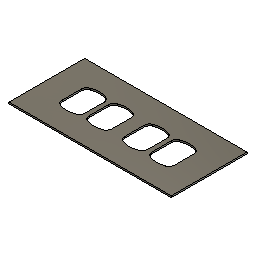
NixieClockFront (Autodesk Fusion 360 design; units mm, degrees)
Autodesk Fusion 360 part; units mm, degrees
sketch "Skizze1" plane through (0, 0, 0) normal (0, 1, 0) x (1, 0, 0)
  line L0 (-60, 12.25) -> (-60, -12.25)
  line L1 (-60, -12.25) -> (-81, -12.25) construction
  line L2 (-81, -12.25) -> (-81, 12.25)
  line L3 (-35, 12.25) -> (-35, -12.25)
  line L4 (-35, -12.25) -> (-56, -12.25) construction
  line L5 (-56, -12.25) -> (-56, 12.25)
  line L6 (-2, 12.25) -> (-2, -12.25)
  line L7 (-2, -12.25) -> (-23, -12.25) construction
  line L8 (-23, -12.25) -> (-23, 12.25)
  line L9 (23, 12.25) -> (23, -12.25)
  line L10 (23, -12.25) -> (2, -12.25) construction
  line L11 (2, -12.25) -> (2, 12.25)
  spline S0 degree 5 poles (-81, 12.25) (-80.58, 12.4586) (-79.74, 12.8575) (-78.48, 13.4013) (-76.8, 14.0152) (-74.7, 14.5849) (-72.6, 14.9392) (-70.5, 15.0605) (-68.4, 14.9392) (-66.3, 14.5849) (-64.2, 14.0152) (-62.52, 13.4013) (-61.26, 12.8575) (-60.42, 12.4586) (-60, 12.25) knots 0 0 0 0 0 0 0.1 0.2 0.3 0.4 0.5 0.6 0.7 0.8 0.9 1 1 1 1 1 1
  spline S1 degree 5 poles (-56, 12.25) (-55.58, 12.4586) (-54.74, 12.8575) (-53.48, 13.4013) (-51.8, 14.0152) (-49.7, 14.5849) (-47.6, 14.9392) (-45.5, 15.0605) (-43.4, 14.9392) (-41.3, 14.5849) (-39.2, 14.0152) (-37.52, 13.4013) (-36.26, 12.8575) (-35.42, 12.4586) (-35, 12.25) knots 0 0 0 0 0 0 0.1 0.2 0.3 0.4 0.5 0.6 0.7 0.8 0.9 1 1 1 1 1 1
  spline S2 degree 5 poles (-23, 12.25) (-22.58, 12.4586) (-21.74, 12.8575) (-20.48, 13.4013) (-18.8, 14.0152) (-16.7, 14.5849) (-14.6, 14.9392) (-12.5, 15.0605) (-10.4, 14.9392) (-8.3, 14.5849) (-6.2, 14.0152) (-4.52, 13.4013) (-3.26, 12.8575) (-2.42, 12.4586) (-2, 12.25) knots 0 0 0 0 0 0 0.1 0.2 0.3 0.4 0.5 0.6 0.7 0.8 0.9 1 1 1 1 1 1
  spline S3 degree 5 poles (2, 12.25) (2.42, 12.4586) (3.26, 12.8575) (4.52, 13.4013) (6.2, 14.0152) (8.3, 14.5849) (10.4, 14.9392) (12.5, 15.0605) (14.6, 14.9392) (16.7, 14.5849) (18.8, 14.0152) (20.48, 13.4013) (21.74, 12.8575) (22.58, 12.4586) (23, 12.25) knots 0 0 0 0 0 0 0.1 0.2 0.3 0.4 0.5 0.6 0.7 0.8 0.9 1 1 1 1 1 1
  spline S4 degree 5 poles (-81, -12.25) (-80.58, -12.4586) (-79.74, -12.8575) (-78.48, -13.4013) (-76.8, -14.0152) (-74.7, -14.5849) (-72.6, -14.9392) (-70.5, -15.0605) (-68.4, -14.9392) (-66.3, -14.5849) (-64.2, -14.0152) (-62.52, -13.4013) (-61.26, -12.8575) (-60.42, -12.4586) (-60, -12.25) knots 0 0 0 0 0 0 0.1 0.2 0.3 0.4 0.5 0.6 0.7 0.8 0.9 1 1 1 1 1 1
  spline S5 degree 5 poles (-56, -12.25) (-55.58, -12.4586) (-54.74, -12.8575) (-53.48, -13.4013) (-51.8, -14.0152) (-49.7, -14.5849) (-47.6, -14.9392) (-45.5, -15.0605) (-43.4, -14.9392) (-41.3, -14.5849) (-39.2, -14.0152) (-37.52, -13.4013) (-36.26, -12.8575) (-35.42, -12.4586) (-35, -12.25) knots 0 0 0 0 0 0 0.1 0.2 0.3 0.4 0.5 0.6 0.7 0.8 0.9 1 1 1 1 1 1
  spline S6 degree 5 poles (-23, -12.25) (-22.58, -12.4586) (-21.74, -12.8575) (-20.48, -13.4013) (-18.8, -14.0152) (-16.7, -14.5849) (-14.6, -14.9392) (-12.5, -15.0605) (-10.4, -14.9392) (-8.3, -14.5849) (-6.2, -14.0152) (-4.52, -13.4013) (-3.26, -12.8575) (-2.42, -12.4586) (-2, -12.25) knots 0 0 0 0 0 0 0.1 0.2 0.3 0.4 0.5 0.6 0.7 0.8 0.9 1 1 1 1 1 1
  spline S7 degree 5 poles (2, -12.25) (2.42, -12.4586) (3.26, -12.8575) (4.52, -13.4013) (6.2, -14.0152) (8.3, -14.5849) (10.4, -14.9392) (12.5, -15.0605) (14.6, -14.9392) (16.7, -14.5849) (18.8, -14.0152) (20.48, -13.4013) (21.74, -12.8575) (22.58, -12.4586) (23, -12.25) knots 0 0 0 0 0 0 0.1 0.2 0.3 0.4 0.5 0.6 0.7 0.8 0.9 1 1 1 1 1 1
  line L12 (-99, 27) -> (-98, 27) construction
  line L13 (-81, 0) -> (-104, 0) construction
  line L14 (23, 0) -> (46, 0) construction
  line L15 (-70.5, 15) -> (-70.5, 35) construction
  line L16 (-70.5, -15) -> (-70.5, -35) construction
  line L17 (-104, 0) -> (-104, -35)
  line L18 (-104, -35) -> (46, -35)
  line L19 (46, -35) -> (46, 35)
  line L20 (46, 35) -> (-104, 35)
  line L21 (-104, 35) -> (-104, 0)
  point P0 (-70.5, 15)
  point P1 (-70.5, -15)
  point P2 (-12.5, 15)
  point P3 (-12.5, -15)
  point P4 (12.5, 15)
  point P5 (12.5, -15)
  point P6 (-45.5, 15)
  point P7 (-45.5, -15)
  point P8 (-45.5, 0)
  point P9 (-12.5, 0)
  point P10 (12.5, 0)
  point P11 (45.5, 0)
  point P12 (70.5, 0.1137)
  dimension "d39" = 21
  dimension "d41" = 21
  dimension "d43" = 21
  dimension "d45" = 21
  dimension "d85" = 4
  dimension "d86" = 12
  dimension "d87" = 4
  dimension "d97" = 104
  dimension "d103" = 23
  dimension "d105" = 20
  dimension "d106" = 20
  dimension "d107" = 21
  dimension "d108" = 21
  dimension "d109" = 21
  dimension "d110" = 21
  dimension "d111" = 23
  constraint parallel L0 L2
  constraint parallel L3 L5
  constraint parallel L6 L8
  constraint parallel L9 L11
  constraint midpoint L2 L13.start
  constraint perpendicular L2 L13
  constraint midpoint L9 L14.start
  constraint perpendicular L9 L14
  constraint coincident P0 L15.start
  constraint coincident P1 L16.start
  constraint perpendicular L13 L17
  constraint perpendicular L16 L18
  constraint perpendicular L14 L19
  constraint perpendicular L15 L20
  constraint perpendicular L13 L21
  measures "d39" distance of L0.end L1.end
  measures "d41" distance of L3.end L4.end
  measures "d43" distance of L6.end L7.end
  measures "d45" distance of L9.end L10.end
  measures "d85" distance of L6 L11
  measures "d86" distance of L3 L8
  measures "d87" distance of L0 L5
  measures "d97" distance of L2.end L9.start
  measures "d103" distance of L13.start L13.end
  measures "d105" distance of P0 L15.end
  measures "d106" distance of P1 L16.end
  measures "d107" distance of L0 L2
  measures "d108" distance of L3 L5
  measures "d109" distance of L6 L8
  measures "d110" distance of L9 L11
  measures "d111" distance of L9.start L19
extrude "Extrusion4" add sketch "Skizze1" along normal blind 1.5
fillet "Abrundung3" radius 5 16 edges at (-81, 0.75, -12.25) (-56, 0.75, -12.25) (-23, 0.75, -12.25) (2, 0.75, -12.25) (-60, 0.75, -12.25) (-35, 0.75, -12.25) (-2, 0.75, -12.25) (23, 0.75, -12.25) (23, 0.75, 12.25) (-2, 0.75, 12.25) (-35, 0.75, 12.25) (-60, 0.75, 12.25) (-81, 0.75, 12.25) (-56, 0.75, 12.25) (-23, 0.75, 12.25) (2, 0.75, 12.25)
